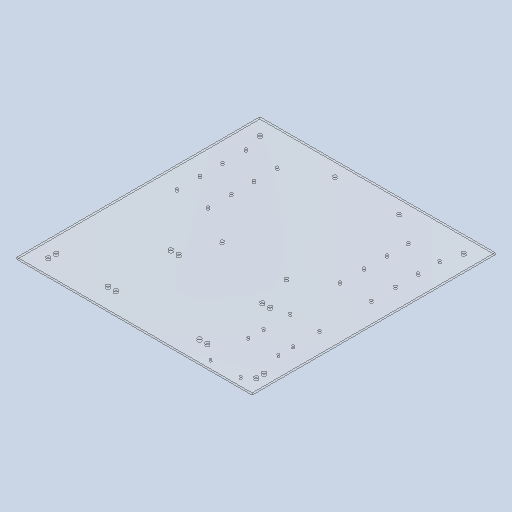
# Autodesk Inventor part: Electronics Base Plate
Saved by Autodesk Inventor 2022 (Build 260153000, 153)
## iProperties
Created: 2022-01-14
Part Number: Electronics Base Plate
Material: Generic
Document SubType Name: Modeling
Designer: merky
Density: 1 g/cm^3
Appearance: Polycarbonate - Clear
Author: merky
Autodesk Inventor part; units mm, degrees
ref_plane "YZ Plane" through (0, 0, 0) normal (1, 0, 0) x (0, 1, 0)
ref_plane "XZ Plane" through (0, 0, 0) normal (0, 1, 0) x (-1, 0, 0)
ref_plane "XY Plane" through (0, 0, 0) normal (0, 0, 1) x (1, 0, 0)
sketch "Sketch1" plane through (0, 0, 0) normal (0, 1, 0) x (-1, 0, 0)
  line L0 (0, 0) -> (381, 0)
  line L1 (381, 0) -> (381, -393.7)
  line L2 (381, -393.7) -> (0, -393.7)
  line L3 (0, -393.7) -> (0, 0)
  dimension "d0" = 381
  dimension "d1" = 393.7
  constraints: 8 end point, 2 parallel, 1 horizontal, 1 perpendicular
  measures "d0" distance of L1.end L2.end
  measures "d1" distance of L0.end L1.end
extrude "Extrusion1" add sketch "Sketch1" along normal blind 3.175
sketch "Sketch2" plane through (0, 3.175, 0) normal (0, 1, 0) x (1, 0, 0)
  circle A0 centre (-32.4064, 14.0157) radius 1.8387
  circle A1 centre (-81.2506, 14.0157) radius 1.8387
  circle A2 centre (-32.4064, 75.0519) radius 1.8387
  circle A3 centre (-81.2506, 75.0519) radius 1.8387
  circle A4 centre (-33.1585, 142.5213) radius 1.905
  circle A5 centre (-33.1562, 99.4683) radius 1.905
  circle A6 centre (-80.9082, 99.4683) radius 1.905
  circle A7 centre (-80.9082, 142.5213) radius 1.905
  circle A8 centre (-33.65, 226.8485) radius 2.3218
  circle A9 centre (-33.65, 226.8485) radius 2.2218
  circle A10 centre (-84.45, 226.8485) radius 2.2218
  circle A11 centre (-33.65, 266.0113) radius 2.2218
  circle A12 centre (-84.45, 266.0113) radius 2.2218
  circle A13 centre (-33.65, 302.8244) radius 2.2218
  circle A14 centre (-84.45, 302.8244) radius 2.2218
  circle A15 centre (-33.65, 337.7088) radius 2.2218
  circle A16 centre (-84.45, 337.7088) radius 2.2218
  circle A17 centre (-132.932, 188.6742) radius 2.667
  circle A18 centre (-237.3259, 188.845) radius 2.667
  circle A19 centre (-132.6339, 370.9444) radius 2.667
  circle A20 centre (-237.0277, 371.1151) radius 2.667
  circle A21 centre (-296.55, 225.4894) radius 2.2218
  circle A22 centre (-347.35, 225.4894) radius 2.2218
  circle A23 centre (-296.55, 262.9154) radius 2.2218
  circle A24 centre (-347.35, 262.9154) radius 2.2218
  circle A25 centre (-296.55, 299.5102) radius 2.2218
  circle A26 centre (-347.35, 299.5102) radius 2.2218
  circle A27 centre (-296.55, 337.2913) radius 2.2218
  circle A28 centre (-347.35, 337.2913) radius 2.2218
  circle A29 centre (-119.0443, 33.9146) radius 3.175
  circle A30 centre (-106.3443, 33.9146) radius 3.175
  circle A31 centre (-254.6769, 33.9146) radius 3.175
  circle A32 centre (-267.3769, 33.9146) radius 3.175
  circle A33 centre (-254.6769, 135.6909) radius 3.175
  circle A34 centre (-267.3769, 135.6909) radius 3.175
  line L0 (0, 393.7) -> (-381, 393.7)
  line L1 (-381, 393.7) -> (-381, 0)
  line L2 (-381, 0) -> (0, 0)
  line L3 (0, 0) -> (0, 393.7)
  line L4 (-381, 393.7) -> (-381, 0) projected
  line L5 (-381, 0) -> (0, 0) projected
  line L6 (-119.0443, 33.9146) -> (-119.0443, 186.178) construction
  circle A35 centre (-119.0443, 135.6909) radius 3.175
  circle A36 centre (-106.3443, 135.6909) radius 3.175
  circle A37 centre (-355.6, 25.4) radius 3.175
  circle A38 centre (-355.6, 368.3) radius 3.175
  circle A39 centre (-25.4, 368.3) radius 3.175
  circle A40 centre (-355.6, 38.1) radius 3.175
  circle A41 centre (-18.7484, 25.4) radius 3.175
  circle A42 centre (-18.7484, 38.1) radius 3.175
  dimension "d13" = 6.35
  dimension "d14" = 6.35
  dimension "d15" = 12.7
  dimension "d16" = 6.35
  dimension "d17" = 6.35
  dimension "d18" = 12.7
  dimension "d19" = 6.35
  dimension "d20" = 6.35
  dimension "d21" = 12.7
  dimension "d22" = 22.5849
  dimension "d23" = 143.9723
  dimension "d24" = 4.4436
  dimension "d25" = 50.8
  dimension "d26" = 33.65
  dimension "d27" = 56.4087
  dimension "d30" = 6.35
  dimension "d31" = 6.35
  dimension "d32" = 12.7
  dimension "d33" = 6.35
  dimension "d34" = 25.4
  dimension "d36" = 25.4
  dimension "d40" = 6.35
  dimension "d41" = 25.4
  dimension "d42" = 25.4
  dimension "d43" = 6.35
  dimension "d44" = 25.4
  dimension "d45" = 25.4
  dimension "d46" = 6.35
  dimension "d47" = 12.7
  dimension "d48" = 6.35
  dimension "d49" = 6.35
  dimension "d50" = 12.7
  constraints: 43 centre point, 10 end point, 3 vertical, 2 horizontal
  measures "d13" diameter of A29
  measures "d14" diameter of A30
  measures "d15" distance of L6.start A30.centre
  measures "d16" diameter of A32
  measures "d17" diameter of A31
  measures "d18" distance of A32.centre A31.centre
  measures "d19" diameter of A34
  measures "d20" diameter of A33
  measures "d21" distance of A34.centre A33.centre
  measures "d22" distance from line of L0 A20.centre
  measures "d23" distance from line of L1 A20.centre
  measures "d24" diameter of A27
  measures "d25" distance of A28.centre A27.centre
  measures "d26" distance from line of L1 A28.centre
  measures "d27" distance from line of L0 A28.centre
  measures "d30" diameter of A35
  measures "d31" diameter of A36
  measures "d32" distance of A35.centre A36.centre
  measures "d33" diameter of A37
  measures "d34" distance from line of A37.centre L4
  measures "d36" distance from line of L2 A37.centre
  measures "d40" diameter of A38
  measures "d41" distance from line of L0 A38.centre
  measures "d42" distance from line of L4 A38.centre
  measures "d43" diameter of A39
  measures "d44" distance from line of A39.centre L3
  measures "d45" distance from line of A39.centre L0
  measures "d46" diameter of A40
  measures "d47" distance of A40.centre A37.centre
  measures "d48" diameter of A41
  measures "d49" diameter of A42
  measures "d50" distance of A42.centre A41.centre
extrude "Extrusion2" cut sketch "Sketch2" against normal through all contours A0 | A1 | A2 | A3 | A4 | A5 | A6 | A7 | A9 | A10 | A11 | A12 | A13 | A14 | A15 | A16 | A17 | A18 | A19 | A20 | A21 | A22 | A23 | A24 | A25 | A26 | A27 | A28 | A29 | A30 | A31 | A32 | A33 | A34 | A35 | A36 | A37 | A38 | A39 | A40 | A41 | A42
body "Solid1"
